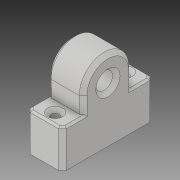
# Autodesk Inventor part: 2316_Pillow Block_V1
Saved by Autodesk Inventor 2020 (Build 240168000, 168)
## iProperties
Created: 2017-07-17
Part Number: 2316_Pillow Block_V1
Material: Generic
Document SubType Name: Modeling
Designer: MPI
Density: 1 g/cm^3
Appearance: Default
Author: MPI
Autodesk Inventor part; units mm, degrees
ref_plane "YZ Plane" through (0, 0, 0) normal (1, 0, 0) x (0, 1, 0)
ref_plane "XZ Plane" through (0, 0, 0) normal (0, 1, 0) x (-1, 0, 0)
ref_plane "XY Plane" through (0, 0, 0) normal (0, 0, 1) x (1, 0, 0)
sketch "Sketch1" plane through (0, 0, 0) normal (1, 0, 0) x (0, 1, 0)
  line L0 (-15.875, 38.1) -> (15.875, 38.1)
  line L1 (15.875, -38.1) -> (-15.875, -38.1)
  line L2 (-15.875, -38.1) -> (-15.875, 38.1)
  line L3 (-15.875, 38.1) -> (15.875, -38.1) construction
  line L4 (15.875, 38.1) -> (-15.875, -38.1) construction
  circle A0 centre (30.2006, 0) radius 14.3256
  line L5 (29.6902, 20.6693) -> (15.875, 20.3282)
  line L6 (30.2006, -20.6756) -> (15.875, -20.6756)
  arc A1 (30.2006, -20.6756) -> (29.6902, 20.6693) centre (30.2006, 0) ccw
  line L7 (15.875, 38.1) -> (15.875, 20.3282)
  line L8 (15.875, -20.6756) -> (15.875, -38.1)
  point P0 (0, 0)
  point P1 (0, 0)
  point P2 (0, 0)
  dimension "d0" = 31.75
  dimension "d2" = 28.6512
  dimension "d4" = 6.35
  dimension "d5" = 1.414
  dimension "d24" = 76.2
  constraints: 18 end point, 4 parallel, 4 perpendicular, 3 midpoint, 3 tangent, 2 centre point, 2 point on circle, 1 coincident, 1 horizontal, 1 horizontal alignment
  measures "d0" distance of L1.start L1.end
  measures "d2" diameter of A0
  measures "d4" radial gap between concentric circles of A0 A1
  measures "d5" angle of L6 L5
  measures "d24" distance between parallel lines of L1 L0
extrude "Extrusion1" add sketch "Sketch1" along normal blind 30
sketch "Sketch2" plane through (30, 0, 0) normal (1, 0, 0) x (0, 0, -1)
  circle A0 centre (0, 30.2006) radius 14.3256 projected
  arc A1 (20.6756, 30.2006) -> (-20.6693, 29.6902) centre (0, 30.2006) ccw projected
  circle A2 centre (0, 30.2006) radius 6.985
  circle A3 centre (0, 30.2006) radius 14.3256
  point P0 (0, 0)
  dimension "d8" = 13.97
  constraints: 2 centre point, 2 coincident
  measures "d8" diameter of A2
extrude "Extrusion2" add sketch "Sketch2" against normal blind 23.396
sketch "Sketch3" plane through (0, 15.875, -20.6756) normal (0, 1, 0) x (1, 0, 0)
  line L0 (30, 0) -> (0, 17.4244)
  line L1 (30, -41.0038) -> (30, -58.7756) projected
  line L2 (0, -41.0038) -> (30, -41.0038) projected
  line L3 (30, -58.7756) -> (0, -41.0038)
  point P0 (0, -20.6756)
  point P1 (15, -49.8897)
  point P2 (15, 8.7122)
  constraints: 4 end point, 2 midpoint
hole "Hole1" at (15, 15.875, 29.2141) at (15, 15.875, -29.3878) direction (0, -1, 0) diameter 6.604 end through all countersink diameter 12.5984 countersink angle 90 clearance for "Flat Head Machine Screw" size "M6" standard "Ansi Metric M Profile"
chamfer "Chamfer1" distance 3.175 angle 45 12 edges at (0, 0, 38.1) (30, 0, 38.1) (0, 0, -38.1) (30, 0, -38.1) (0, 50.8746, 0.2552) (0, 23.0378, -20.6756) (0, 22.7826, 20.4987) (30, 50.8746, 0.2552) (30, 22.7826, 20.4987) (30, 23.0378, -20.6756) (30, 30.2006, 6.985) (6.604, 30.2006, 6.985)
chamfer "Chamfer2" distance 1.5875 angle 45 11 edges at (0, 15.875, -27.8003) (15, 15.875, -38.1) (30, 15.875, -27.8003) (30, 15.875, 27.6266) (28.4125, 15.875, 36.5125) (15, 15.875, 38.1) (1.5875, 15.875, 36.5125) (0, 15.875, 27.6266) (1.5875, 15.875, -36.5125) (28.4125, 15.875, -36.5125) (0, 15.875, 0)
body "Solid1"
